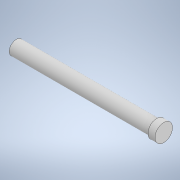
# Autodesk Inventor part: fakeM4BoltLonger
Saved by Autodesk Inventor 2020 (Build 240168000, 168)
## iProperties
Created: 2019-11-14
Part Number: fakeM4BoltLonger
Material: Generic
Document SubType Name: Modeling
Designer: bzs3334
Density: 1 g/cm^3
Appearance: Default
Author: bzs3334
Autodesk Inventor part; units mm, degrees
ref_plane "YZ Plane" through (0, 0, 0) normal (1, 0, 0) x (0, 1, 0)
ref_plane "XZ Plane" through (0, 0, 0) normal (0, 1, 0) x (-1, 0, 0)
ref_plane "XY Plane" through (0, 0, 0) normal (0, 0, 1) x (1, 0, 0)
sketch "Sketch1" plane through (0, 0, 0) normal (1, 0, 0) x (0, 1, 0)
  circle A0 centre (0, 0) radius 2
  dimension "d0" = 4
  constraints: 1 centre point, 1 coincident
  measures "d0" diameter of A0
extrude "Extrusion1" add sketch "Sketch1" along normal blind 40
sketch "Sketch2" plane through (40, 0, 0) normal (1, 0, 0) x (0, 0, -1)
  circle A0 centre (0, 0) radius 2 projected
  circle A1 centre (0, 0) radius 2.5
  dimension "d3" = 5
  constraints: 1 centre point, 1 coincident
  measures "d3" diameter of A1
extrude "Extrusion2" add sketch "Sketch2" along normal blind 2 contours A0 | A1
body "Solid1"
